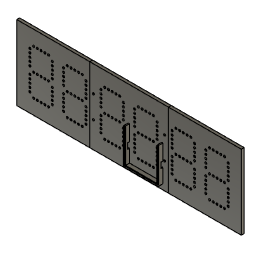
led6digitCAD (Autodesk Fusion 360 design; units mm, degrees)
Autodesk Fusion 360 part; units mm, degrees
sketch "Esquisse1" plane through (0, 0, 0) normal (0, 1, 0) x (1, 0, 0)
  line L0 (0, 0) -> (600, 0)
  line L1 (600, 0) -> (600, -200)
  line L2 (600, -200) -> (0, -200)
  line L3 (0, -200) -> (0, 0)
  line L4 (0, -100) -> (20, -100) construction
  line L5 (400, -100) -> (490, -100) construction
  line L6 (490, -100) -> (580, -100) construction
  line L7 (40, -35) -> (90, -35)
  line L8 (90, -35) -> (90, -45)
  line L9 (90, -45) -> (40, -45)
  line L10 (40, -45) -> (40, -35)
  line L11 (40, -45) -> (30, -45)
  line L12 (30, -45) -> (30, -95)
  line L13 (30, -95) -> (40, -95)
  line L14 (40, -95) -> (40, -45)
  line L15 (90, -45) -> (100, -45)
  line L16 (100, -45) -> (100, -95)
  line L17 (100, -95) -> (90, -95)
  line L18 (90, -95) -> (90, -45)
  line L19 (90, -105) -> (100, -105)
  line L20 (100, -105) -> (100, -155)
  line L21 (100, -155) -> (90, -155)
  line L22 (90, -155) -> (90, -105)
  line L23 (90, -105) -> (40, -105)
  line L24 (40, -105) -> (40, -95)
  line L25 (40, -95) -> (90, -95)
  line L26 (90, -95) -> (90, -105)
  line L27 (40, -105) -> (30, -105)
  line L28 (30, -105) -> (30, -155)
  line L29 (30, -155) -> (40, -155)
  line L30 (40, -155) -> (40, -105)
  line L31 (40, -155) -> (90, -155)
  line L32 (90, -155) -> (90, -165)
  line L33 (90, -165) -> (40, -165)
  line L34 (40, -165) -> (40, -155)
  line L35 (130, -95) -> (180, -95)
  line L36 (180, -95) -> (180, -105)
  line L37 (180, -105) -> (130, -105)
  line L38 (130, -105) -> (130, -95)
  line L39 (120, -105) -> (120, -155)
  line L40 (120, -155) -> (130, -155)
  line L41 (130, -105) -> (120, -105)
  line L42 (130, -155) -> (130, -105)
  line L43 (130, -155) -> (180, -155)
  line L44 (180, -155) -> (180, -165)
  line L45 (130, -165) -> (130, -155)
  line L46 (180, -165) -> (130, -165)
  line L47 (180, -105) -> (190, -105)
  line L48 (190, -155) -> (180, -155)
  line L49 (180, -155) -> (180, -105)
  line L50 (190, -105) -> (190, -155)
  line L51 (180, -45) -> (190, -45)
  line L52 (190, -95) -> (180, -95)
  line L53 (180, -95) -> (180, -45)
  line L54 (190, -45) -> (190, -95)
  line L55 (130, -45) -> (130, -35)
  line L56 (180, -35) -> (180, -45)
  line L57 (130, -35) -> (180, -35)
  line L58 (130, -45) -> (120, -45)
  line L59 (120, -95) -> (130, -95)
  line L60 (120, -45) -> (120, -95)
  line L61 (180, -45) -> (130, -45)
  line L62 (130, -95) -> (130, -45)
  line L63 (320, -155) -> (320, -105)
  line L64 (370, -95) -> (370, -105)
  line L65 (320, -165) -> (320, -155)
  line L66 (370, -155) -> (370, -105)
  line L67 (370, -35) -> (370, -45)
  line L68 (370, -95) -> (370, -45)
  line L69 (230, -45) -> (230, -35)
  line L70 (230, -155) -> (280, -155)
  line L71 (280, -95) -> (280, -105)
  line L72 (290, -155) -> (280, -155)
  line L73 (280, -155) -> (280, -105)
  line L74 (380, -155) -> (370, -155)
  line L75 (320, -95) -> (370, -95)
  line L76 (370, -45) -> (320, -45)
  line L77 (370, -155) -> (370, -165)
  line L78 (380, -105) -> (380, -155)
  line L79 (320, -35) -> (370, -35)
  line L80 (320, -45) -> (320, -35)
  line L81 (370, -105) -> (380, -105)
  line L82 (230, -105) -> (220, -105)
  line L83 (370, -165) -> (320, -165)
  line L84 (320, -105) -> (320, -95)
  line L85 (310, -105) -> (310, -155)
  line L86 (370, -105) -> (320, -105)
  line L87 (380, -45) -> (380, -95)
  line L88 (230, -45) -> (220, -45)
  line L89 (230, -95) -> (280, -95)
  line L90 (380, -95) -> (370, -95)
  line L91 (280, -95) -> (280, -45)
  line L92 (230, -105) -> (230, -95)
  line L93 (280, -105) -> (230, -105)
  line L94 (280, -35) -> (280, -45)
  line L95 (290, -105) -> (290, -155)
  line L96 (230, -95) -> (230, -45)
  line L97 (280, -155) -> (280, -165)
  line L98 (290, -45) -> (290, -95)
  line L99 (220, -95) -> (230, -95)
  line L100 (320, -155) -> (370, -155)
  line L101 (310, -45) -> (310, -95)
  line L102 (230, -165) -> (230, -155)
  line L103 (280, -45) -> (230, -45)
  line L104 (280, -165) -> (230, -165)
  line L105 (280, -45) -> (290, -45)
  line L106 (290, -95) -> (280, -95)
  line L107 (230, -35) -> (280, -35)
  line L108 (230, -155) -> (230, -105)
  line L109 (220, -155) -> (230, -155)
  line L110 (280, -105) -> (290, -105)
  line L111 (310, -95) -> (320, -95)
  line L112 (320, -95) -> (320, -45)
  line L113 (320, -45) -> (310, -45)
  line L114 (370, -45) -> (380, -45)
  line L115 (320, -105) -> (310, -105)
  line L116 (310, -155) -> (320, -155)
  line L117 (220, -105) -> (220, -155)
  line L118 (220, -95) -> (220, -45)
  line L119 (560, -165) -> (510, -165)
  line L120 (500, -95) -> (510, -95)
  line L121 (510, -105) -> (500, -105)
  line L122 (510, -45) -> (500, -45)
  line L123 (500, -155) -> (510, -155)
  line L124 (560, -95) -> (560, -105)
  line L125 (500, -45) -> (500, -95)
  line L126 (510, -155) -> (560, -155)
  line L127 (510, -105) -> (510, -95)
  line L128 (570, -155) -> (560, -155)
  line L129 (410, -95) -> (420, -95)
  line L130 (480, -155) -> (470, -155)
  line L131 (470, -155) -> (470, -105)
  line L132 (470, -105) -> (420, -105)
  line L133 (470, -35) -> (470, -45)
  line L134 (470, -165) -> (420, -165)
  line L135 (470, -155) -> (470, -165)
  line L136 (420, -165) -> (420, -155)
  line L137 (470, -45) -> (480, -45)
  line L138 (420, -105) -> (420, -95)
  line L139 (470, -95) -> (470, -105)
  line L140 (500, -105) -> (500, -155)
  line L141 (560, -105) -> (510, -105)
  line L142 (560, -105) -> (570, -105)
  line L143 (560, -45) -> (570, -45)
  line L144 (480, -45) -> (480, -95)
  line L145 (420, -95) -> (420, -45)
  line L146 (510, -165) -> (510, -155)
  line L147 (470, -95) -> (470, -45)
  line L148 (570, -105) -> (570, -155)
  line L149 (570, -95) -> (560, -95)
  line L150 (510, -35) -> (560, -35)
  line L151 (560, -155) -> (560, -165)
  line L152 (510, -155) -> (510, -105)
  line L153 (420, -155) -> (420, -105)
  line L154 (560, -155) -> (560, -105)
  line L155 (420, -105) -> (410, -105)
  line L156 (510, -45) -> (510, -35)
  line L157 (470, -105) -> (480, -105)
  line L158 (420, -45) -> (410, -45)
  line L159 (480, -95) -> (470, -95)
  line L160 (480, -105) -> (480, -155)
  line L161 (470, -45) -> (420, -45)
  line L162 (420, -155) -> (470, -155)
  line L163 (560, -45) -> (510, -45)
  line L164 (510, -95) -> (560, -95)
  line L165 (560, -95) -> (560, -45)
  line L166 (510, -95) -> (510, -45)
  line L167 (410, -105) -> (410, -155)
  line L168 (420, -45) -> (420, -35)
  line L169 (420, -35) -> (470, -35)
  line L170 (570, -45) -> (570, -95)
  line L171 (420, -95) -> (470, -95)
  line L172 (410, -45) -> (410, -95)
  line L173 (410, -155) -> (420, -155)
  line L174 (560, -35) -> (560, -45)
  line L175 (200, -75) -> (210, -75)
  line L176 (210, -75) -> (210, -65)
  line L177 (210, -65) -> (200, -65)
  line L178 (200, -65) -> (200, -75)
  line L179 (200, -135) -> (210, -135)
  line L180 (210, -135) -> (210, -125)
  line L181 (210, -125) -> (200, -125)
  line L182 (200, -125) -> (200, -135)
  line L183 (390, -135) -> (400, -135)
  line L184 (400, -135) -> (400, -125)
  line L185 (390, -125) -> (390, -135)
  line L186 (400, -125) -> (390, -125)
  line L187 (390, -75) -> (400, -75)
  line L188 (400, -75) -> (400, -65)
  line L189 (390, -65) -> (390, -75)
  line L190 (400, -65) -> (390, -65)
  dimension "d1" = 600
  dimension "d2" = 200
  dimension "d3" = 20
  dimension "d10" = 90
  dimension "d11" = 90
  dimension "d14" = 190
  dimension "d15" = 0
  constraint horizontal L0
  constraint vertical L1
  constraint horizontal L2
  constraint vertical L3
  constraint coincident L0.start L3.end
  constraint midpoint L3 L4.start
  constraint perpendicular L1 L4
  constraint horizontal L7
  constraint vertical L8
  constraint horizontal L9
  constraint vertical L10
  constraint horizontal L11
  constraint vertical L12
  constraint horizontal L13
  constraint vertical L14
  constraint horizontal L15
  constraint vertical L16
  constraint horizontal L17
  constraint vertical L18
  constraint horizontal L19
  constraint vertical L20
  constraint horizontal L21
  constraint vertical L22
  constraint horizontal L23
  constraint vertical L24
  constraint horizontal L25
  constraint vertical L26
  constraint horizontal L27
  constraint vertical L28
  constraint horizontal L29
  constraint vertical L30
  constraint horizontal L31
  constraint vertical L32
  constraint horizontal L33
  constraint vertical L34
  constraint horizontal L57
  constraint vertical L56
  constraint horizontal L61
  constraint vertical L55
  constraint horizontal L58
  constraint vertical L60
  constraint horizontal L59
  constraint vertical L62
  constraint horizontal L51
  constraint vertical L54
  constraint horizontal L52
  constraint vertical L53
  constraint horizontal L47
  constraint vertical L50
  constraint horizontal L48
  constraint vertical L49
  constraint horizontal L37
  constraint vertical L38
  constraint horizontal L35
  constraint vertical L36
  constraint horizontal L41
  constraint vertical L39
  constraint horizontal L40
  constraint vertical L42
  constraint horizontal L43
  constraint vertical L44
  constraint horizontal L46
  constraint vertical L45
  constraint horizontal L107
  constraint vertical L94
  constraint horizontal L103
  constraint vertical L69
  constraint horizontal L88
  constraint horizontal L99
  constraint vertical L96
  constraint horizontal L105
  constraint vertical L98
  constraint horizontal L106
  constraint vertical L91
  constraint horizontal L110
  constraint vertical L95
  constraint horizontal L72
  constraint vertical L73
  constraint horizontal L93
  constraint vertical L92
  constraint horizontal L89
  constraint vertical L71
  constraint horizontal L82
  constraint horizontal L109
  constraint vertical L108
  constraint horizontal L70
  constraint vertical L97
  constraint horizontal L104
  constraint vertical L102
  constraint horizontal L79
  constraint vertical L67
  constraint horizontal L76
  constraint vertical L80
  constraint horizontal L113
  constraint vertical L101
  constraint horizontal L111
  constraint vertical L112
  constraint horizontal L114
  constraint vertical L87
  constraint horizontal L90
  constraint vertical L68
  constraint horizontal L81
  constraint vertical L78
  constraint horizontal L74
  constraint vertical L66
  constraint horizontal L86
  constraint vertical L84
  constraint horizontal L75
  constraint vertical L64
  constraint horizontal L115
  constraint vertical L85
  constraint horizontal L116
  constraint vertical L63
  constraint horizontal L100
  constraint vertical L77
  constraint horizontal L83
  constraint vertical L65
  constraint perpendicular L109 L117
  constraint perpendicular L2 L118
  constraint horizontal L169
  constraint vertical L133
  constraint horizontal L161
  constraint vertical L168
  constraint horizontal L158
  constraint vertical L172
  constraint horizontal L129
  constraint vertical L145
  constraint horizontal L137
  constraint vertical L144
  constraint horizontal L159
  constraint vertical L147
  constraint horizontal L157
  constraint vertical L160
  constraint horizontal L130
  constraint vertical L131
  constraint horizontal L132
  constraint vertical L138
  constraint horizontal L171
  constraint vertical L139
  constraint horizontal L155
  constraint vertical L167
  constraint horizontal L173
  constraint vertical L153
  constraint horizontal L162
  constraint vertical L135
  constraint horizontal L134
  constraint vertical L136
  constraint horizontal L150
  constraint vertical L174
  constraint horizontal L163
  constraint vertical L156
  constraint horizontal L122
  constraint vertical L125
  constraint horizontal L120
  constraint vertical L166
  constraint horizontal L143
  constraint vertical L170
  constraint horizontal L149
  constraint vertical L165
  constraint horizontal L142
  constraint vertical L148
  constraint horizontal L128
  constraint vertical L154
  constraint horizontal L141
  constraint vertical L127
  constraint horizontal L164
  constraint vertical L124
  constraint horizontal L121
  constraint vertical L140
  constraint horizontal L123
  constraint vertical L152
  constraint horizontal L126
  constraint vertical L151
  constraint horizontal L119
  constraint vertical L146
  constraint horizontal L175
  constraint vertical L176
  constraint horizontal L177
  constraint vertical L178
  constraint horizontal L179
  constraint vertical L180
  constraint horizontal L181
  constraint vertical L182
  measures "d1" distance of L0.start L0.end
  measures "d2" distance of L0.start L2.end
  measures "d3" distance of L4.start L4.end
  measures "d10" distance of L5.end L5.start
  measures "d11" distance of L5.end L6.end
extrude "Extrusion1" add sketch "Esquisse1" along normal blind 5 contours L0 L1 L2 L3 | L9 L14 L18 L25 | L22 L23 L30 L31 | L35 L53 L61 L62 | L37 L42 L43 L49 | L63 L66 L86 L100 | L68 L75 L76 L112 | L89 L91 L96 L103 | L70 L73 L93 L108 | L126 L141 L152 L154 | L163 L164 L165 L166 | L145 L147 L161 L171 | L131 L132 L153 L162 makes body 1
sketch "Esquisse2" plane through (0, 0, 0) normal (0, -1, 0) x (1, 0, 0)
  line L0 (400, 65) -> (390, 65)
  line L1 (390, 65) -> (390, 75)
  line L2 (390, 75) -> (400, 75)
  line L3 (400, 75) -> (400, 65)
  line L4 (40, 45) -> (30, 45)
  line L5 (30, 45) -> (30, 95)
  line L6 (30, 95) -> (40, 95)
  line L7 (40, 95) -> (40, 105)
  line L8 (40, 105) -> (30, 105)
  line L9 (30, 105) -> (30, 155)
  line L10 (30, 155) -> (40, 155)
  line L11 (40, 155) -> (40, 165)
  line L12 (40, 165) -> (90, 165)
  line L13 (90, 165) -> (90, 155)
  line L14 (90, 155) -> (100, 155)
  line L15 (100, 155) -> (100, 105)
  line L16 (100, 105) -> (90, 105)
  line L17 (90, 105) -> (90, 95)
  line L18 (90, 95) -> (100, 95)
  line L19 (100, 95) -> (100, 45)
  line L20 (100, 45) -> (90, 45)
  line L21 (90, 45) -> (90, 35)
  line L22 (90, 35) -> (40, 35)
  line L23 (40, 35) -> (40, 45)
  line L24 (320, 105) -> (310, 105)
  line L25 (310, 105) -> (310, 155)
  line L26 (310, 155) -> (320, 155)
  line L27 (320, 155) -> (320, 165)
  line L28 (320, 165) -> (370, 165)
  line L29 (370, 165) -> (370, 155)
  line L30 (370, 155) -> (380, 155)
  line L31 (380, 155) -> (380, 105)
  line L32 (380, 105) -> (370, 105)
  line L33 (370, 105) -> (370, 95)
  line L34 (370, 95) -> (380, 95)
  line L35 (380, 95) -> (380, 45)
  line L36 (380, 45) -> (370, 45)
  line L37 (370, 45) -> (370, 35)
  line L38 (370, 35) -> (320, 35)
  line L39 (320, 35) -> (320, 45)
  line L40 (320, 45) -> (310, 45)
  line L41 (310, 45) -> (310, 95)
  line L42 (310, 95) -> (320, 95)
  line L43 (320, 95) -> (320, 105)
  line L44 (230, 105) -> (220, 105)
  line L45 (220, 105) -> (220, 155)
  line L46 (220, 155) -> (230, 155)
  line L47 (230, 155) -> (230, 165)
  line L48 (230, 165) -> (280, 165)
  line L49 (280, 165) -> (280, 155)
  line L50 (280, 155) -> (290, 155)
  line L51 (290, 155) -> (290, 105)
  line L52 (290, 105) -> (280, 105)
  line L53 (280, 105) -> (280, 95)
  line L54 (280, 95) -> (290, 95)
  line L55 (290, 95) -> (290, 45)
  line L56 (290, 45) -> (280, 45)
  line L57 (280, 45) -> (280, 35)
  line L58 (280, 35) -> (230, 35)
  line L59 (230, 35) -> (230, 45)
  line L60 (230, 45) -> (220, 45)
  line L61 (220, 45) -> (220, 95)
  line L62 (220, 95) -> (230, 95)
  line L63 (230, 95) -> (230, 105)
  line L64 (420, 105) -> (410, 105)
  line L65 (410, 105) -> (410, 155)
  line L66 (410, 155) -> (420, 155)
  line L67 (420, 155) -> (420, 165)
  line L68 (420, 165) -> (470, 165)
  line L69 (470, 165) -> (470, 155)
  line L70 (470, 155) -> (480, 155)
  line L71 (480, 155) -> (480, 105)
  line L72 (480, 105) -> (470, 105)
  line L73 (470, 105) -> (470, 95)
  line L74 (470, 95) -> (480, 95)
  line L75 (480, 95) -> (480, 45)
  line L76 (480, 45) -> (470, 45)
  line L77 (470, 45) -> (470, 35)
  line L78 (470, 35) -> (420, 35)
  line L79 (420, 35) -> (420, 45)
  line L80 (420, 45) -> (410, 45)
  line L81 (410, 45) -> (410, 95)
  line L82 (410, 95) -> (420, 95)
  line L83 (420, 95) -> (420, 105)
  line L84 (400, 125) -> (390, 125)
  line L85 (390, 125) -> (390, 135)
  line L86 (390, 135) -> (400, 135)
  line L87 (400, 135) -> (400, 125)
  line L88 (510, 45) -> (500, 45)
  line L89 (500, 45) -> (500, 95)
  line L90 (500, 95) -> (510, 95)
  line L91 (510, 95) -> (510, 105)
  line L92 (510, 105) -> (500, 105)
  line L93 (500, 105) -> (500, 155)
  line L94 (500, 155) -> (510, 155)
  line L95 (510, 155) -> (510, 165)
  line L96 (510, 165) -> (560, 165)
  line L97 (560, 165) -> (560, 155)
  line L98 (560, 155) -> (570, 155)
  line L99 (570, 155) -> (570, 105)
  line L100 (570, 105) -> (560, 105)
  line L101 (560, 105) -> (560, 95)
  line L102 (560, 95) -> (570, 95)
  line L103 (570, 95) -> (570, 45)
  line L104 (570, 45) -> (560, 45)
  line L105 (560, 45) -> (560, 35)
  line L106 (560, 35) -> (510, 35)
  line L107 (510, 35) -> (510, 45)
  line L108 (200, 65) -> (200, 75)
  line L109 (200, 75) -> (210, 75)
  line L110 (210, 75) -> (210, 65)
  line L111 (210, 65) -> (200, 65)
  line L112 (130, 45) -> (120, 45)
  line L113 (120, 45) -> (120, 95)
  line L114 (120, 95) -> (130, 95)
  line L115 (130, 95) -> (130, 105)
  line L116 (130, 105) -> (120, 105)
  line L117 (120, 105) -> (120, 155)
  line L118 (120, 155) -> (130, 155)
  line L119 (130, 155) -> (130, 165)
  line L120 (130, 165) -> (180, 165)
  line L121 (180, 165) -> (180, 155)
  line L122 (180, 155) -> (190, 155)
  line L123 (190, 155) -> (190, 105)
  line L124 (190, 105) -> (180, 105)
  line L125 (180, 105) -> (180, 95)
  line L126 (180, 95) -> (190, 95)
  line L127 (190, 95) -> (190, 45)
  line L128 (190, 45) -> (180, 45)
  line L129 (180, 45) -> (180, 35)
  line L130 (180, 35) -> (130, 35)
  line L131 (130, 35) -> (130, 45)
  line L132 (200, 125) -> (200, 135)
  line L133 (200, 135) -> (210, 135)
  line L134 (210, 135) -> (210, 125)
  line L135 (210, 125) -> (200, 125)
  line L136 (600, 200) -> (0, 200)
  line L137 (0, 200) -> (0, 0)
  line L138 (0, 0) -> (600, 0)
  line L139 (600, 0) -> (600, 200)
  circle A0 centre (35, 90) radius 2.75
  circle A1 centre (35, 80) radius 2.75
  circle A2 centre (35, 70) radius 2.75
  circle A3 centre (35, 60) radius 2.75
  circle A4 centre (35, 50) radius 2.75
  circle A5 centre (95, 90) radius 2.75
  circle A6 centre (95, 80) radius 2.75
  circle A7 centre (95, 70) radius 2.75
  circle A8 centre (95, 60) radius 2.75
  circle A9 centre (95, 50) radius 2.75
  circle A10 centre (35, 150) radius 2.75
  circle A11 centre (35, 140) radius 2.75
  circle A12 centre (35, 130) radius 2.75
  circle A13 centre (35, 110) radius 2.75
  circle A14 centre (35, 120) radius 2.75
  circle A15 centre (95, 150) radius 2.75
  circle A16 centre (95, 140) radius 2.75
  circle A17 centre (95, 130) radius 2.75
  circle A18 centre (95, 110) radius 2.75
  circle A19 centre (95, 120) radius 2.75
  circle A20 centre (45, 40) radius 2.75
  circle A21 centre (55, 40) radius 2.75
  circle A22 centre (65, 40) radius 2.75
  circle A23 centre (75, 40) radius 2.75
  circle A24 centre (85, 40) radius 2.75
  circle A25 centre (85, 100) radius 2.75
  circle A26 centre (45, 100) radius 2.75
  circle A27 centre (55, 100) radius 2.75
  circle A28 centre (65, 100) radius 2.75
  circle A29 centre (75, 100) radius 2.75
  circle A30 centre (85, 160) radius 2.75
  circle A31 centre (45, 160) radius 2.75
  circle A32 centre (55, 160) radius 2.75
  circle A33 centre (65, 160) radius 2.75
  circle A34 centre (75, 160) radius 2.75
  circle A35 centre (145, 160) radius 2.75
  circle A36 centre (185, 110) radius 2.75
  circle A37 centre (125, 150) radius 2.75
  circle A38 centre (125, 80) radius 2.75
  circle A39 centre (135, 160) radius 2.75
  circle A40 centre (125, 140) radius 2.75
  circle A41 centre (185, 80) radius 2.75
  circle A42 centre (185, 150) radius 2.75
  circle A43 centre (185, 140) radius 2.75
  circle A44 centre (185, 120) radius 2.75
  circle A45 centre (125, 110) radius 2.75
  circle A46 centre (185, 60) radius 2.75
  circle A47 centre (125, 70) radius 2.75
  circle A48 centre (165, 40) radius 2.75
  circle A49 centre (125, 120) radius 2.75
  circle A50 centre (145, 100) radius 2.75
  circle A51 centre (155, 40) radius 2.75
  circle A52 centre (125, 90) radius 2.75
  circle A53 centre (125, 130) radius 2.75
  circle A54 centre (135, 40) radius 2.75
  circle A55 centre (125, 50) radius 2.75
  circle A56 centre (155, 160) radius 2.75
  circle A57 centre (175, 40) radius 2.75
  circle A58 centre (185, 50) radius 2.75
  circle A59 centre (185, 70) radius 2.75
  circle A60 centre (125, 60) radius 2.75
  circle A61 centre (185, 130) radius 2.75
  circle A62 centre (185, 90) radius 2.75
  circle A63 centre (175, 160) radius 2.75
  circle A64 centre (145, 40) radius 2.75
  circle A65 centre (155, 100) radius 2.75
  circle A66 centre (135, 100) radius 2.75
  circle A67 centre (175, 100) radius 2.75
  circle A68 centre (165, 160) radius 2.75
  circle A69 centre (165, 100) radius 2.75
  circle A70 centre (245, 160) radius 2.75
  circle A71 centre (285, 110) radius 2.75
  circle A72 centre (225, 150) radius 2.75
  circle A73 centre (225, 80) radius 2.75
  circle A74 centre (235, 160) radius 2.75
  circle A75 centre (225, 140) radius 2.75
  circle A76 centre (285, 80) radius 2.75
  circle A77 centre (285, 150) radius 2.75
  circle A78 centre (285, 140) radius 2.75
  circle A79 centre (285, 120) radius 2.75
  circle A80 centre (225, 110) radius 2.75
  circle A81 centre (285, 60) radius 2.75
  circle A82 centre (225, 70) radius 2.75
  circle A83 centre (265, 40) radius 2.75
  circle A84 centre (225, 120) radius 2.75
  circle A85 centre (245, 100) radius 2.75
  circle A86 centre (255, 40) radius 2.75
  circle A87 centre (225, 90) radius 2.75
  circle A88 centre (225, 130) radius 2.75
  circle A89 centre (235, 40) radius 2.75
  circle A90 centre (225, 50) radius 2.75
  circle A91 centre (255, 160) radius 2.75
  circle A92 centre (275, 40) radius 2.75
  circle A93 centre (285, 50) radius 2.75
  circle A94 centre (285, 70) radius 2.75
  circle A95 centre (225, 60) radius 2.75
  circle A96 centre (285, 130) radius 2.75
  circle A97 centre (285, 90) radius 2.75
  circle A98 centre (275, 160) radius 2.75
  circle A99 centre (245, 40) radius 2.75
  circle A100 centre (255, 100) radius 2.75
  circle A101 centre (235, 100) radius 2.75
  circle A102 centre (275, 100) radius 2.75
  circle A103 centre (265, 160) radius 2.75
  circle A104 centre (265, 100) radius 2.75
  circle A105 centre (335, 160) radius 2.75
  circle A106 centre (375, 110) radius 2.75
  circle A107 centre (315, 150) radius 2.75
  circle A108 centre (315, 80) radius 2.75
  circle A109 centre (325, 160) radius 2.75
  circle A110 centre (315, 140) radius 2.75
  circle A111 centre (375, 80) radius 2.75
  circle A112 centre (375, 150) radius 2.75
  circle A113 centre (375, 140) radius 2.75
  circle A114 centre (375, 120) radius 2.75
  circle A115 centre (315, 110) radius 2.75
  circle A116 centre (375, 60) radius 2.75
  circle A117 centre (315, 70) radius 2.75
  circle A118 centre (355, 40) radius 2.75
  circle A119 centre (315, 120) radius 2.75
  circle A120 centre (335, 100) radius 2.75
  circle A121 centre (345, 40) radius 2.75
  circle A122 centre (315, 90) radius 2.75
  circle A123 centre (315, 130) radius 2.75
  circle A124 centre (325, 40) radius 2.75
  circle A125 centre (315, 50) radius 2.75
  circle A126 centre (345, 160) radius 2.75
  circle A127 centre (365, 40) radius 2.75
  circle A128 centre (375, 50) radius 2.75
  circle A129 centre (375, 70) radius 2.75
  circle A130 centre (315, 60) radius 2.75
  circle A131 centre (375, 130) radius 2.75
  circle A132 centre (375, 90) radius 2.75
  circle A133 centre (365, 160) radius 2.75
  circle A134 centre (335, 40) radius 2.75
  circle A135 centre (345, 100) radius 2.75
  circle A136 centre (325, 100) radius 2.75
  circle A137 centre (365, 100) radius 2.75
  circle A138 centre (355, 160) radius 2.75
  circle A139 centre (355, 100) radius 2.75
  circle A140 centre (435, 160) radius 2.75
  circle A141 centre (475, 110) radius 2.75
  circle A142 centre (415, 150) radius 2.75
  circle A143 centre (415, 80) radius 2.75
  circle A144 centre (425, 160) radius 2.75
  circle A145 centre (415, 140) radius 2.75
  circle A146 centre (475, 80) radius 2.75
  circle A147 centre (475, 150) radius 2.75
  circle A148 centre (475, 140) radius 2.75
  circle A149 centre (475, 120) radius 2.75
  circle A150 centre (415, 110) radius 2.75
  circle A151 centre (475, 60) radius 2.75
  circle A152 centre (415, 70) radius 2.75
  circle A153 centre (455, 40) radius 2.75
  circle A154 centre (415, 120) radius 2.75
  circle A155 centre (435, 100) radius 2.75
  circle A156 centre (445, 40) radius 2.75
  circle A157 centre (415, 90) radius 2.75
  circle A158 centre (415, 130) radius 2.75
  circle A159 centre (425, 40) radius 2.75
  circle A160 centre (415, 50) radius 2.75
  circle A161 centre (445, 160) radius 2.75
  circle A162 centre (465, 40) radius 2.75
  circle A163 centre (475, 50) radius 2.75
  circle A164 centre (475, 70) radius 2.75
  circle A165 centre (415, 60) radius 2.75
  circle A166 centre (475, 130) radius 2.75
  circle A167 centre (475, 90) radius 2.75
  circle A168 centre (465, 160) radius 2.75
  circle A169 centre (435, 40) radius 2.75
  circle A170 centre (445, 100) radius 2.75
  circle A171 centre (425, 100) radius 2.75
  circle A172 centre (465, 100) radius 2.75
  circle A173 centre (455, 160) radius 2.75
  circle A174 centre (455, 100) radius 2.75
  circle A175 centre (525, 160) radius 2.75
  circle A176 centre (565, 110) radius 2.75
  circle A177 centre (505, 150) radius 2.75
  circle A178 centre (505, 80) radius 2.75
  circle A179 centre (515, 160) radius 2.75
  circle A180 centre (505, 140) radius 2.75
  circle A181 centre (565, 80) radius 2.75
  circle A182 centre (565, 150) radius 2.75
  circle A183 centre (565, 140) radius 2.75
  circle A184 centre (565, 120) radius 2.75
  circle A185 centre (505, 110) radius 2.75
  circle A186 centre (565, 60) radius 2.75
  circle A187 centre (505, 70) radius 2.75
  circle A188 centre (545, 40) radius 2.75
  circle A189 centre (505, 120) radius 2.75
  circle A190 centre (525, 100) radius 2.75
  circle A191 centre (535, 40) radius 2.75
  circle A192 centre (505, 90) radius 2.75
  circle A193 centre (505, 130) radius 2.75
  circle A194 centre (515, 40) radius 2.75
  circle A195 centre (505, 50) radius 2.75
  circle A196 centre (535, 160) radius 2.75
  circle A197 centre (555, 40) radius 2.75
  circle A198 centre (565, 50) radius 2.75
  circle A199 centre (565, 70) radius 2.75
  circle A200 centre (505, 60) radius 2.75
  circle A201 centre (565, 130) radius 2.75
  circle A202 centre (565, 90) radius 2.75
  circle A203 centre (555, 160) radius 2.75
  circle A204 centre (525, 40) radius 2.75
  circle A205 centre (535, 100) radius 2.75
  circle A206 centre (515, 100) radius 2.75
  circle A207 centre (555, 100) radius 2.75
  circle A208 centre (545, 160) radius 2.75
  circle A209 centre (545, 100) radius 2.75
  circle A210 centre (205, 70) radius 2.75
  circle A211 centre (205, 130) radius 2.75
  circle A212 centre (395, 70) radius 2.75
  circle A213 centre (395, 130) radius 2.75
  point P0 (185, 70)
  dimension "d19" = 5.5
  dimension "d28" = 5.5
  dimension "d34" = 5.5
  dimension "d35" = 5.5
  dimension "d36" = 5.5
  dimension "d45" = 5.5
  dimension "d46" = 5.5
  dimension "d47" = 5.5
  dimension "d48" = 5.5
  dimension "d49" = 5.5
  dimension "d50" = 5.5
  dimension "d51" = 5.5
  dimension "d52" = 5.5
  dimension "d53" = 5.5
  dimension "d54" = 5.5
  dimension "d55" = 5.5
  dimension "d56" = 5.5
  dimension "d57" = 5.5
  dimension "d58" = 5.5
  dimension "d59" = 5.5
  dimension "d60" = 5.5
  dimension "d61" = 5.5
  dimension "d62" = 5.5
  dimension "d63" = 5.5
  dimension "d64" = 5.5
  dimension "d65" = 5.5
  dimension "d66" = 5.5
  dimension "d67" = 5.5
  dimension "d68" = 5.5
  dimension "d69" = 5.5
  measures "d19" diameter of A0
  measures "d28" diameter of A5
  measures "d34" diameter of A10
  measures "d35" diameter of A15
  measures "d36" diameter of A20
  measures "d45" diameter of A52
  measures "d46" diameter of A62
  measures "d47" diameter of A37
  measures "d48" diameter of A42
  measures "d49" diameter of A54
  measures "d50" diameter of A87
  measures "d51" diameter of A97
  measures "d52" diameter of A72
  measures "d53" diameter of A77
  measures "d54" diameter of A89
  measures "d55" diameter of A122
  measures "d56" diameter of A132
  measures "d57" diameter of A107
  measures "d58" diameter of A112
  measures "d59" diameter of A124
  measures "d60" diameter of A157
  measures "d61" diameter of A167
  measures "d62" diameter of A142
  measures "d63" diameter of A147
  measures "d64" diameter of A159
  measures "d65" diameter of A192
  measures "d66" diameter of A202
  measures "d67" diameter of A177
  measures "d68" diameter of A182
  measures "d69" diameter of A194
extrude "Extrusion2" add sketch "Esquisse2" along normal blind 2.5 separate body contours L0 L1 L2 L3 | L4 L5 L6 L7 L8 L9 L10 L11 L12 L13 L14 L15 L16 L17 L18 L19 L20 L21 L22 L23 | L24 L25 L26 L27 L28 L29 L30 L31 L32 L33 L34 L35 L36 L37 L38 L39 L40 L41 L42 L43 | L44 L45 L46 L47 L48 L49 L50 L51 L52 L53 L54 L55 L56 L57 L58 L59 L60 L61 L62 L63 | L64 L65 L66 L67 L68 L69 L70 L71 L72 L73 L74 L75 L76 L77 L78 L79 L80 L81 L82 L83 | L84 L85 L86 L87 | L88 L89 L90 L91 L92 L93 L94 L95 L96 L97 L98 L99 L100 L101 L102 L103 L104 L105 L106 L107 | L108 L109 L110 L111 | L112 L113 L114 L115 L116 L117 L118 L119 L120 L121 L122 L123 L124 L125 L126 L127 L128 L129 L130 L131 | L132 L133 L134 L135 | L136 L137 L138 L139 makes body 2
combine "Combiner1" operation add target body 1 tool bodies 2
extrude "Extrusion3" cut 1 faces at (200, 0, 200) along direction (0, 0, -1) blind 0.5 on bodies 1 bodies 1
extrude "Extrusion4" cut 1 faces at (400, 0, 0) along direction (0, 0, 1) blind 0.5 on bodies 1 bodies 1
ref_plane "Plan de construction1" through (195, 1.25, 100) normal (-1, 0, 0) x (0, 0, 1)
ref_plane "Plan de construction2" through (405, 1.25, 100) normal (-1, 0, 0) x (0, 0, 1)
split "Scinder1" by plane through (405, 1.25, 100) normal (-1, 0, 0) and through (195, 1.25, 100) normal (-1, 0, 0) bodies 1 makes body 3 at (93.3333, -2.5, 12.75) makes body 4 at (291.7625, -2.5, 187.245)
ref_plane "Plan de construction3" through (300, -22.5, 100) normal (0, -1, 0) x (1, 0, 0)
sketch "Esquisse3" plane through (300, -22.5, 100) normal (0, -1, 0) x (1, 0, 0)
  line L0 (-50, 70) -> (40, 70)
  line L1 (40, 70) -> (40, -20)
  line L2 (40, -20) -> (-50, -20)
  line L3 (-50, -20) -> (-50, 70)
  dimension "d79" = 90
  dimension "d80" = 90
  constraint horizontal L0
  constraint vertical L1
  constraint horizontal L2
  constraint vertical L3
  measures "d79" distance of L0.start L0.end
  measures "d80" distance of L0.start L2.end
extrude "Extrusion5" add sketch "Esquisse3" along normal blind 1.6 separate body makes body 5
sketch "Esquisse4" plane through (0, 0, 170) normal (0, 0, 1) x (-1, 0, 0)
  line L0 (-340, 22.5) -> (-250, 22.5)
  line L1 (-250, 22.5) -> (-250, 24.1)
  line L2 (-250, 24.1) -> (-340, 24.1)
  line L3 (-340, 24.1) -> (-340, 22.5)
  line L4 (-340.25, 22.25) -> (-340.25, 24.35)
  line L5 (-249.75, 24.35) -> (-249.75, 22.25)
  line L6 (-249.25, 24.85) -> (-249.25, 21.75)
  line L7 (-340.75, 21.75) -> (-340.75, 24.85)
  line L8 (-250, 22.5) -> (-252, 22.5) construction
  line L9 (-252, 22.25) -> (-252, 21.75)
  line L10 (-252, 24.35) -> (-252, 24.85)
  line L11 (-295, 22.5) -> (-295, 24.1) construction
  line L12 (-338, 22.25) -> (-338, 21.75)
  line L13 (-338, 24.35) -> (-338, 24.85)
  line L14 (-249.75, 22.25) -> (-252, 22.25)
  line L15 (-338, 22.25) -> (-340.25, 22.25)
  line L16 (-249.25, 21.75) -> (-252, 21.75)
  line L17 (-338, 21.75) -> (-340.75, 21.75)
  line L18 (-340.75, 24.85) -> (-338, 24.85)
  line L19 (-252, 24.85) -> (-249.25, 24.85)
  line L20 (-340.25, 24.35) -> (-338, 24.35)
  line L21 (-252, 24.35) -> (-249.75, 24.35)
  dimension "d85" = 90.5
  dimension "d86" = 2.1
  constraint horizontal L14
  constraint vertical L4
  constraint horizontal L20
  constraint vertical L5
  constraint coincident L0.end L1.start
  constraint coincident L0 L8.end
  constraint perpendicular L1 L8
  constraint coincident L10.start L20
  constraint coincident L10.end L18
  constraint perpendicular L10 L18
  constraint midpoint L0 L11.start
  constraint midpoint L2 L11.end
  constraint symmetric L9.end L11 L12.end
  constraint symmetric L9.start L11 L12.start
  constraint symmetric L10.start L11 L13.start
  constraint symmetric L10.end L11 L13.end
  constraint collinear L14 L15
  constraint parallel L18 L20
  constraint parallel L5 L6
  constraint parallel L4 L7
  constraint collinear L16 L17
  constraint collinear L18 L19
  constraint collinear L20 L21
  measures "d85" distance of L5.end L4.start
  measures "d86" distance of L5.end L5.start
extrude "Extrusion6" add sketch "Esquisse4" against normal blind 90.25 separate body contours L4 L7 L12 L13 L15 L17 L18 L20 | L5 L6 L9 L10 L14 L16 L19 L21 makes body 6 at (340.75, -22.7833, 139.9167) makes body 7 at (249.25, -23.8167, 109.8333)
sketch "Esquisse5" plane through (0, 0, 79.75) normal (0, 0, -1) x (1, 0, 0)
  line L0 (252, 24.35) -> (252, 24.85)
  line L1 (252, 24.85) -> (249.25, 24.85)
  line L2 (249.25, 24.85) -> (249.25, 21.75)
  line L3 (249.25, 21.75) -> (252, 21.75)
  line L4 (252, 21.75) -> (252, 22.25)
  line L5 (252, 22.25) -> (249.75, 22.25)
  line L6 (249.75, 22.25) -> (249.75, 24.35)
  line L7 (249.75, 24.35) -> (252, 24.35)
  line L8 (249.25, 24.85) -> (340.75, 24.85)
  line L9 (340.75, 24.85) -> (340.75, 21.75)
  line L10 (340.75, 21.75) -> (249.25, 21.75)
  line L11 (249.25, 21.75) -> (249.25, 24.85)
  constraint horizontal L8
  constraint vertical L9
  constraint horizontal L10
  constraint vertical L11
  constraint coincident L1.end L2.start
extrude "Extrusion7" add sketch "Esquisse5" along normal blind 2.5 bodies 6 7
move_body "Déplacer1" bodies 5 6 to x (1, 0, 0) y (0, 1, 0) z (0, 0, 1) at (0, -132.22, 0)
extrude "Extrusion8" add 3 faces at (338.9167, -153.97, 139.9167) (310.25, -153.97, 78.0833) (250.1667, -153.97, 109) along direction (0, 1, 0) blind 10 on bodies 6 bodies 6
extrude "Extrusion9" add 2 faces at (250.3333, -147.47, 170) (339.6667, -147.47, 170) along direction (0, 0, 1) blind 1 on bodies 6 bodies 6
move_body "Déplacer2" bodies 5 6 to x (1, 0, 0) y (0, 1, 0) z (0, 0, 1) at (55, 0, 0)
move_body "Déplacer3" bodies 5 6 to x (1, 0, 0) y (0, 1, 0) z (0, 0, 1) at (9.25, 141.47, -76.75)
move_body "Déplacer4" bodies 5 6 to x (1, 0, 0) y (0, 1, 0) z (0, 0, 1) at (-15, 0, 15)
sketch "Esquisse6" plane through (390, 0, 0) normal (1, 0, 0) x (0, 1, 0)
  line L0 (-15.6, 109.25) -> (-15.6, 18)
  line L1 (-15.6, 18) -> (-15.6, 15.5)
  line L2 (-15.6, 15.5) -> (-12.5, 15.5)
  line L3 (-12.5, 15.5) -> (-2.5, 15.5)
  line L4 (-2.5, 15.5) -> (-2.5, 18)
  line L5 (-2.5, 18) -> (-2.5, 109.25)
  line L6 (-2.5, 109.25) -> (-15.6, 109.25)
  line L7 (-7.5, 52.5) -> (-2.5, 52.5)
  line L8 (-2.5, 52.5) -> (-2.5, 67.5)
  line L9 (-2.5, 67.5) -> (-7.5, 67.5)
  line L10 (-7.5, 67.5) -> (-7.5, 52.5)
  dimension "d96" = 5
  dimension "d97" = 15
  constraint horizontal L7
  constraint vertical L8
  constraint horizontal L9
  constraint vertical L10
  measures "d96" distance of L7.start L7.end
  measures "d97" distance of L7.start L9.end
extrude "Extrusion10" cut sketch "Esquisse6" against normal blind 121.5 contours L5 L7 L8 L9 L10 bodies 6
extrude "Extrusion11" add 1 faces at (298.5, -8.5333, 95.3333) along direction (-1, 0, 0) blind 0.5 on bodies 6 bodies 6
extrude "Extrusion12" add 2 faces at (390, -10.2, 16.3333) (390, -8.5333, 95.3333) along direction (1, 0, 0) blind 0.5 on bodies 6 bodies 6
delete_face "DeleteFace1" 1 faces at (300.3333, -15.6, 48.4167) on bodies 6
extrude "Extrusion13" add 1 faces at (329.9167, -11.2333, 15.5) along direction (0, 0, -1) blind 0.75 on bodies 6 bodies 6
sketch "Esquisse7" plane through (0, 0, 18) normal (0, 0, 1) x (-1, 0, 0)
  line L0 (-387.25, 15.6) -> (-387.25, 15.1)
  line L1 (-387.25, 15.1) -> (-389.5, 15.1)
  line L2 (-389.5, 15.1) -> (-389.5, 13)
  line L3 (-389.5, 13) -> (-387.25, 13)
  line L4 (-387.25, 13) -> (-387.25, 2.5)
  line L5 (-387.25, 2.5) -> (-301.25, 2.5)
  line L6 (-301.25, 2.5) -> (-301.25, 13)
  line L7 (-301.25, 13) -> (-299, 13)
  line L8 (-299, 13) -> (-299, 15.1)
  line L9 (-299, 15.1) -> (-301.25, 15.1)
  line L10 (-301.25, 15.1) -> (-301.25, 15.6)
  line L11 (-301.25, 15.6) -> (-387.25, 15.6)
  line L12 (-299, 13) -> (-389.5, 13)
  line L13 (-389.5, 13) -> (-389.5, 15.1)
  line L14 (-389.5, 15.1) -> (-299, 15.1)
  line L15 (-299, 15.1) -> (-299, 13)
  constraint horizontal L12
  constraint vertical L13
  constraint horizontal L14
  constraint vertical L15
  constraint coincident L1.end L2.start
  constraint coincident L7.end L8.start
extrude "Extrusion14" cut sketch "Esquisse7" against normal blind 0.5 contours L1 L2 L3 L7 L8 L9 L12 L13 L14 L15 bodies 6
sketch "Esquisse8" plane through (0, -14.85, 0) normal (0, -1, 0) x (1, 0, 0)
  line L0 (299.25, 18.25) -> (389.25, 18.25)
  line L1 (389.25, 18.25) -> (389.25, 108.25)
  line L2 (389.25, 108.25) -> (299.25, 108.25)
  line L3 (299.25, 108.25) -> (299.25, 18.25)
  line L4 (381.63, 46.02) -> (381.63, 35.86) construction
  line L5 (381.63, 35.86) -> (381.63, 25.7) construction
  line L6 (381.63, 35.86) -> (389.25, 35.86) construction
  line L7 (384.63, 49.02) -> (378.63, 49.02)
  line L8 (378.63, 49.02) -> (378.63, 43.02)
  line L9 (378.63, 43.02) -> (384.63, 43.02)
  line L10 (384.63, 43.02) -> (384.63, 49.02)
  line L11 (384.63, 49.02) -> (378.63, 43.02) construction
  line L12 (378.63, 49.02) -> (384.63, 43.02) construction
  line L13 (384.63, 38.86) -> (378.63, 38.86)
  line L14 (378.63, 38.86) -> (378.63, 32.86)
  line L15 (378.63, 32.86) -> (384.63, 32.86)
  line L16 (384.63, 32.86) -> (384.63, 38.86)
  line L17 (384.63, 38.86) -> (378.63, 32.86) construction
  line L18 (378.63, 38.86) -> (384.63, 32.86) construction
  line L19 (384.63, 28.7) -> (378.63, 28.7)
  line L20 (378.63, 28.7) -> (378.63, 22.7)
  line L21 (378.63, 22.7) -> (384.63, 22.7)
  line L22 (384.63, 22.7) -> (384.63, 28.7)
  line L23 (384.63, 28.7) -> (378.63, 22.7) construction
  line L24 (378.63, 28.7) -> (384.63, 22.7) construction
  point P0 (381.63, 46.02)
  point P1 (381.63, 35.86)
  point P2 (381.63, 25.7)
  dimension "d110" = 10.16
  dimension "d111" = 10.16
  dimension "d112" = 6
  dimension "d113" = 6
  dimension "d114" = 6
  dimension "d115" = 6
  dimension "d116" = 6
  dimension "d117" = 6
  constraint coincident L1 L6.end
  constraint perpendicular L1 L6
  constraint horizontal L7
  constraint perpendicular L7 L8
  constraint parallel L7 L9
  constraint parallel L8 L10
  constraint coincident L11 P0
  constraint coincident L12 P0
  constraint coincident P0 L4.start
  constraint horizontal L13
  constraint perpendicular L13 L14
  constraint parallel L13 L15
  constraint parallel L14 L16
  constraint coincident L17 P1
  constraint coincident L18 P1
  constraint coincident P1 L4.end
  constraint horizontal L19
  constraint perpendicular L19 L20
  constraint parallel L19 L21
  constraint parallel L20 L22
  constraint coincident L23 P2
  constraint coincident L24 P2
  constraint coincident P2 L5.end
  measures "d110" distance of P0 P1
  measures "d111" distance of P1 P2
  measures "d112" distance of L8.end L9.end
  measures "d113" distance of L7.end L8.end
  measures "d114" distance of L14.end L15.end
  measures "d115" distance of L13.end L14.end
  measures "d116" distance of L20.end L21.end
  measures "d117" distance of L19.end L20.end
extrude "Extrusion15" add sketch "Esquisse8" along normal blind 3.5 contours L7 L8 L9 L10 | L13 L14 L15 L16 | L19 L20 L21 L22 bodies 5
sketch "Esquisse9" plane through (0, -18.35, 0) normal (0, -1, 0) x (1, 0, 0)
  line L0 (384.63, 43.02) -> (384.63, 49.02)
  line L1 (384.63, 49.02) -> (378.63, 49.02)
  line L2 (378.63, 49.02) -> (378.63, 43.02)
  line L3 (378.63, 43.02) -> (384.63, 43.02)
  circle A0 centre (381.63, 46.02) radius 1.75
  dimension "d120" = 3.5
  measures "d120" diameter of A0
extrude "Extrusion16" add sketch "Esquisse9" along normal blind 0.8 contours A0 bodies 5
sketch "Esquisse10" plane through (0, -18.35, 0) normal (0, -1, 0) x (1, 0, 0)
  line L0 (384.63, 32.86) -> (384.63, 38.86)
  line L1 (384.63, 38.86) -> (378.63, 38.86)
  line L2 (378.63, 38.86) -> (378.63, 32.86)
  line L3 (378.63, 32.86) -> (384.63, 32.86)
  circle A0 centre (381.63, 35.86) radius 1.75
  dimension "d123" = 3.5
  measures "d123" diameter of A0
extrude "Extrusion17" add sketch "Esquisse10" along normal blind 0.8 contours A0 bodies 5
sketch "Esquisse11" plane through (0, -18.35, 0) normal (0, -1, 0) x (1, 0, 0)
  line L0 (384.63, 22.7) -> (384.63, 28.7)
  line L1 (384.63, 28.7) -> (378.63, 28.7)
  line L2 (378.63, 28.7) -> (378.63, 22.7)
  line L3 (378.63, 22.7) -> (384.63, 22.7)
  circle A0 centre (381.63, 25.7) radius 1.75
  dimension "d126" = 3.5
  measures "d126" diameter of A0
extrude "Extrusion18" add sketch "Esquisse11" along normal blind 0.8 contours A0 bodies 5
ref_plane "Plan de construction4" through (381.63, -18.7891, 47.77) normal (0, 0, 1) x (1, 0, 0)
ref_plane "Plan de construction5" through (381.63, -18.7891, 46.02) normal (0, 0, 1) x (1, 0, 0)
sketch "Esquisse12" plane through (381.63, -18.7891, 46.02) normal (0, 0, 1) x (1, 0, 0)
  line L0 (-2, -0.5) -> (-2, -0.2)
  line L1 (-2, -0.2) -> (-4.5, -0.2)
  line L2 (0, -0.5) -> (0, -4.5)
  line L3 (0, -4.5) -> (-4, -4.5)
  line L4 (-2, -0.5) -> (0, -0.5)
  line L5 (-4.5, -0.2) -> (-4.5, -1)
  line L6 (-4.5, -1) -> (-4, -1)
  line L7 (-4, -1) -> (-4, -4.5)
  dimension "d131" = 4
  dimension "d132" = 4
  dimension "d133" = 0.5
  constraint vertical L0
  constraint perpendicular L0 L1
  constraint perpendicular L1 L2
  constraint perpendicular L2 L3
  constraint perpendicular L2 L4
  constraint perpendicular L5 L6
  constraint perpendicular L6 L7
  constraint perpendicular L3 L7
  measures "d131" distance of L2.start L2.end
  measures "d132" distance of L2.end L3.end
  measures "d133" distance of L5.end L6.end
revolve "Révolution1" add sketch "Esquisse12" angle 360 about axis through (381.63, -18.35, 46.02) along (0, 1, 0) separate body makes body 8
copy_body "CopyPasteBodies1" bodies 8 makes body 9
move_body "Déplacer5" bodies 9 to x (1, 0, 0) y (0, 1, 0) z (0, 0, 1) at (0, 0, -10.16)
copy_body "CopyPasteBodies2" bodies 9 makes body 10
move_body "Déplacer6" bodies 10 to x (1, 0, 0) y (0, 1, 0) z (0, 0, 1) at (0, 0, -10.16)
combine "Combiner2" operation add target body 6 tool bodies 4
hidden bodies 5 8 9 10
equation "d86 = 1.850 mm + 0.25 mm"
equation "d104 = 3.25 mm - 2.5 mm"
equation "d121 = 4.3 mm - 3.5 mm"
equation "d124 = 4.3 mm - 3.5 mm"
equation "d127 = 4.3 mm - 3.5 mm"
equation "d130 = ( -3.5 / 2 ) * 1 mm"
